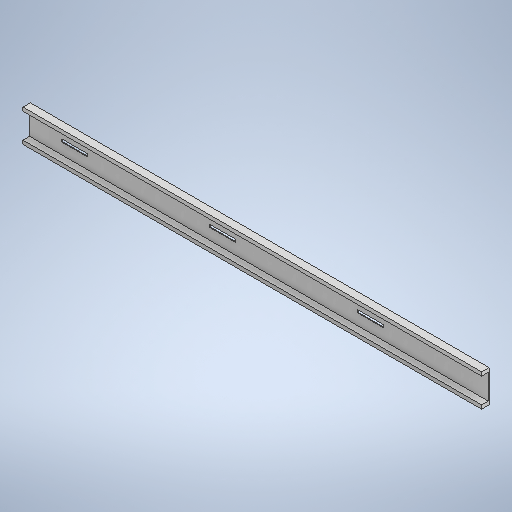
# Autodesk Inventor part: Bracket holder
Saved by Autodesk Inventor 2025.1 (Build 291241020, 241B)
## iProperties
Created: 2024-09-24
Part Number: Bracket holder
Material: Generic
Document SubType Name: Modeling
Designer: jjk
Density: 1 g/cm^3
Appearance: Default
Author: jjk
Autodesk Inventor part; units mm, degrees
ref_plane "YZ Plane" through (0, 0, 0) normal (1, 0, 0) x (0, 1, 0)
ref_plane "XZ Plane" through (0, 0, 0) normal (0, 1, 0) x (-1, 0, 0)
ref_plane "XY Plane" through (0, 0, 0) normal (0, 0, 1) x (1, 0, 0)
sketch "Sketch1" plane through (0, 0, 0) normal (0, 0, 1) x (1, 0, 0)
  line L0 (0, 0) -> (157.48, 0)
  line L1 (157.48, 0) -> (157.48, 11.1125)
  line L2 (157.48, 11.1125) -> (0, 11.1125)
  line L3 (0, 11.1125) -> (0, 0)
  line L4 (0, 11.1125) -> (157.48, 11.1125)
  line L5 (157.48, 11.1125) -> (157.48, 9.8425)
  line L6 (157.48, 9.8425) -> (0, 9.8425)
  line L7 (0, 9.8425) -> (0, 11.1125)
  line L8 (0, 0) -> (157.48, 0)
  line L9 (157.48, 0) -> (157.48, 1.27)
  line L10 (157.48, 1.27) -> (0, 1.27)
  line L11 (0, 1.27) -> (0, 0)
  line L12 (11.0159, 5.08) -> (19.9525, 5.08)
  line L13 (19.9525, 5.08) -> (19.9525, 6.0325)
  line L14 (19.9525, 6.0325) -> (11.0159, 6.0325)
  line L15 (11.0159, 6.0325) -> (11.0159, 5.08)
  line L16 (70.7525, 5.08) -> (70.7525, 6.0325)
  line L17 (70.7525, 6.0325) -> (61.8159, 6.0325)
  line L18 (61.8159, 5.08) -> (70.7525, 5.08)
  line L19 (61.8159, 6.0325) -> (61.8159, 5.08)
  line L20 (121.5525, 5.08) -> (121.5525, 6.0325)
  line L21 (121.5525, 6.0325) -> (112.6159, 6.0325)
  line L22 (112.6159, 5.08) -> (121.5525, 5.08)
  line L23 (112.6159, 6.0325) -> (112.6159, 5.08)
  point P0 (39.5656, 5.08)
  point P1 (47.7905, 6.0325)
  point P2 (98.5905, 6.0325)
  point P3 (90.3656, 5.08)
  point P4 (149.3905, 6.0325)
  point P5 (141.1656, 5.08)
  point P6 (0, 9.8425)
  point P7 (0, 1.27)
  dimension "d0" = 157.48
  dimension "d1" = 11.1125
  dimension "d2" = 1.27
  dimension "d3" = 1.27
  dimension "d4" = 3.81
  dimension "d5" = 3.81
  dimension "d6" = 8.9366
  dimension "d9" = 50.8
  constraints: 48 end point, 8 parallel, 8 point on line, 5 horizontal, 4 perpendicular, 20 other
  measures "d0" distance of L1.end L2.end
  measures "d1" distance of L0.end L1.end
  measures "d2" distance between parallel lines of L2 L6
  measures "d3" distance between parallel lines of L0 L10
  measures "d4" distance between parallel lines of L10 L12
  measures "d5" distance between parallel lines of L6 L14
  measures "d6" distance between parallel lines of L13 L15
  measures "d9" distance of L13.end L16.end
extrude "Extrusion1" add sketch "Sketch1" along normal blind 2.54 contours L3 L10 L1 L0 | L3 L2 L1 L6
extrude "Extrusion2" add sketch "Sketch1" along normal blind 0.254 contours L3 L6 L1 L10
body "Solid1"
